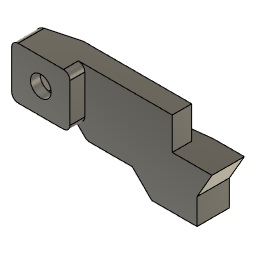
Omnivore adapter plate (Autodesk Fusion 360 design; units mm, degrees)
Autodesk Fusion 360 part; units mm, degrees
sketch "Sketch1" plane through (0, 0, 0) normal (0, 1, 0) x (1, 0, 0)
  line L0 (4.5, -4) -> (-4.5, -4)
  line L1 (-4.5, -4) -> (-4.5, 4)
  line L2 (-4.5, 4) -> (4.5, 4)
  line L3 (4.5, 4) -> (4.5, -4)
  line L4 (4.5, -4) -> (-4.5, 4) construction
  line L5 (-4.5, -4) -> (4.5, 4) construction
  dimension "d164" = 9
  dimension "d165" = 8
  constraint horizontal L0
  constraint perpendicular L0 L1
  constraint parallel L0 L2
  constraint parallel L1 L3
  constraint coincident L4 origin
  constraint coincident L5 origin
  measures "d164" distance of L1.end L2.end
  measures "d165" distance of L0.start L2.end
extrude "Extrude1" add sketch "Sketch1" along normal blind 2.3 makes body 1
fillet "Fillet1" radius 1 2 edges at (-4.5, 1.15, 4) (-4.5, 1.15, -4) on bodies 1
sketch "Sketch2" plane through (0, 2.3, 0) normal (0, 1, 0) x (-1, 0, 0)
  line L0 (-4.5, -4) -> (3.5, -4)
  arc A0 (3.5, -4) -> (4.5, -3) centre (3.5, -3) ccw
  line L1 (4.5, -3) -> (4.5, 3)
  arc A1 (4.5, 3) -> (3.5, 4) centre (3.5, 3) ccw
  line L2 (3.5, 4) -> (-4.5, 4)
  line L3 (-4.5, 4) -> (-4.5, -4)
  line L4 (-3.4641, 0) -> (-1.7321, -3)
  line L5 (-1.7321, -3) -> (1.7321, -3)
  line L6 (1.7321, -3) -> (3.4641, 0)
  line L7 (3.4641, 0) -> (1.7321, 3)
  line L8 (1.7321, 3) -> (-1.7321, 3)
  line L9 (-1.7321, 3) -> (-3.4641, 0)
  dimension "d170" = 6
  constraint horizontal L5
  measures "d170" distance of L4 L7
extrude "Extrude2" cut sketch "Sketch2" against normal up to surface (2.3 mm away) contours L4 L5 L6 L7 L8 L9 bodies 1
sketch "Sketch8" plane through (0, 2.3, 0) normal (0, 1, 0) x (-1, 0, 0)
  line L0 (-1.7321, -3) -> (-3.4641, 0)
  line L1 (-3.4641, 0) -> (-1.7321, 3)
  line L2 (-1.7321, 3) -> (1.7321, 3)
  line L3 (1.7321, 3) -> (3.4641, 0)
  line L4 (3.4641, 0) -> (1.7321, -3)
  line L5 (1.7321, -3) -> (-1.7321, -3)
  arc A0 (3.5, -4) -> (4.5, -3) centre (3.5, -3) ccw
  line L6 (4.5, -3) -> (4.5, 3)
  arc A1 (4.5, 3) -> (3.5, 4) centre (3.5, 3) ccw
  line L7 (3.5, 4) -> (-4.5, 4)
  line L8 (-4.5, 4) -> (-4.5, -4)
  line L9 (-4.5, -4) -> (3.5, -4)
extrude "Extrude6" add sketch "Sketch8" along normal blind 3 separate body makes body 2
sketch "Sketch19" plane through (0, 0, 0) normal (0, -1, 0) x (-1, 0, 0)
  line L0 (3.4641, 0) -> (1.7321, -3)
  line L1 (1.7321, -3) -> (-1.7321, -3)
  line L2 (-1.7321, -3) -> (-3.4641, 0)
  line L3 (-3.4641, 0) -> (-1.7321, 3)
  line L4 (-1.7321, 3) -> (1.7321, 3)
  line L5 (1.7321, 3) -> (3.4641, 0)
  line L6 (-4.5, -4) -> (3.5, -4)
  arc A0 (3.5, -4) -> (4.5, -3) centre (3.5, -3) ccw
  line L7 (4.5, -3) -> (4.5, 3)
  arc A1 (4.5, 3) -> (3.5, 4) centre (3.5, 3) ccw
  line L8 (3.5, 4) -> (-4.5, 4)
  line L9 (-4.5, 4) -> (-4.5, -4)
  line L10 (1.7321, -3) -> (3.4641, 0)
  line L11 (3.4641, 0) -> (1.7321, 3)
  line L12 (1.7321, 3) -> (-1.7321, 3)
  line L13 (-1.7321, 3) -> (-3.4641, 0)
  line L14 (-3.4641, 0) -> (-1.7321, -3)
  line L15 (-1.7321, -3) -> (1.7321, -3)
  circle A2 centre (0, 0) radius 1.6
  line L16 (3.4641, 0) -> (1.7321, -3)
  line L17 (1.7321, -3) -> (-1.7321, -3)
  line L18 (-1.7321, -3) -> (-3.4641, 0)
  line L19 (-3.4641, 0) -> (-1.7321, 3)
  line L20 (-1.7321, 3) -> (1.7321, 3)
  line L21 (1.7321, 3) -> (3.4641, 0)
  arc A3 (4.5, 3) -> (3.5, 4) centre (3.5, 3) ccw
  line L22 (3.5, 4) -> (-4.5, 4)
  line L23 (-4.5, 4) -> (-4.5, -4)
  line L24 (-4.5, -4) -> (3.5, -4)
  arc A4 (3.5, -4) -> (4.5, -3) centre (3.5, -3) ccw
  line L25 (4.5, -3) -> (4.5, 3)
  dimension "d231" = 3.2
  constraint collinear L4 L12
  constraint coincident L3.end L4.start
  constraint coincident L4.end L5.start
  constraint coincident A2.centre origin
  measures "d231" diameter of A2
extrude "Extrude14" add sketch "Sketch19" against normal blind 1.5 contours L0 L1 L2 L3 L4 L5 L10 L11 L12 L13 L14 L15 L16 L17 L18 L19 L20 L21 bodies 1
fillet "Fillet3" radius 1 2 edges at (4.5, 1.15, 4) (4.5, 1.15, -4) on bodies 1
sketch "Sketch11" plane through (4.5, 0, 0) normal (1, 0, 0) x (0, 1, 0)
  line L0 (2.3, 4) -> (2.3, -4)
  line L1 (2.3, -4) -> (5.3, -4)
  line L2 (5.3, -4) -> (5.3, 4)
  line L3 (5.3, 4) -> (2.3, 4)
extrude "Extrude7" add sketch "Sketch11" along normal blind 13.5 bodies 2 1
sketch "Sketch12" plane through (0, 0, -4) normal (0, 0, -1) x (1, 0, 0)
  line L0 (18, -2.3) -> (3.5, -2.3)
  line L1 (-3.5, 0) -> (-3.5, -5.3)
  line L2 (-3.5, -5.3) -> (18, -5.3)
  line L3 (18, -5.3) -> (18, -2.3)
  line L4 (18, -5.3) -> (2.83, -5.3)
  line L5 (2.83, -5.3) -> (2.83, -2.3)
  line L6 (2.83, -2.3) -> (18, -2.3)
  line L7 (18, -2.3) -> (18, -5.3)
  line L8 (3.5, -2.3) -> (3.5, 0)
  line L9 (3.5, 0) -> (-3.5, 0)
  line L10 (-4.5, 0) -> (-4.5, -5.3) construction
  dimension "d242" = 7.33
  constraint horizontal L4
  constraint vertical L5
  constraint horizontal L6
  constraint vertical L7
  constraint coincident L0 L5.end
  constraint coincident L2.end L3.start
  measures "d242" distance of L5 L10
extrude "Extrude8" add sketch "Sketch12" along normal blind 10 from surface at -8 contours L0 L2 L3 L4 L5 L6 L7 bodies 2
chamfer "Chamfer1" distance 2 angle 45 1 edges at (2.83, 3.8, -6) on bodies 2
fillet "Fillet6" radius 1 1 edges at (4.83, 3.8, -6) on bodies 2
ref_plane "WorkPlane1" through (18, 3.8, -6) normal (-0.707107, 0, 0.707107) x (0, -1, 0)
sketch "Sketch17" plane through (0, 5.3, 0) normal (0, 1, 0) x (-1, 0, 0)
  line L0 (-2.83, -4) -> (3.5, -4)
  arc A0 (3.5, -4) -> (4.5, -3) centre (3.5, -3) ccw
  line L1 (4.5, -3) -> (4.5, 3)
  arc A1 (4.5, 3) -> (3.5, 4) centre (3.5, 3) ccw
  line L2 (3.5, 4) -> (-18, 4)
  line L3 (-18, 4) -> (-18, -6)
  line L4 (-18, -6) -> (-5.2442, -6)
  line L5 (-4.5371, -5.7071) -> (-2.83, -4)
  line L6 (-18, -1) -> (-24.1394, -1)
  line L7 (-24.1394, -1) -> (-21.83, -5)
  line L8 (-21.83, -5) -> (-21.83, -9)
  line L9 (-21.83, -9) -> (-11.83, -9)
  line L10 (-11.83, -9) -> (-11.83, -6)
  arc A2 (-5.2442, -6) -> (-4.5371, -5.7071) centre (-5.2442, -5) ccw
  line L11 (-2.83, -1.0983) -> (-2.83, 1.0983) construction
  line L12 (-2.83, 1.0983) -> (-1.7321, 3) construction
  line L13 (-1.7321, 3) -> (1.7321, 3) construction
  line L14 (1.7321, 3) -> (3.4641, 0) construction
  line L15 (3.4641, 0) -> (1.7321, -3) construction
  line L16 (1.7321, -3) -> (-1.7321, -3) construction
  line L17 (-1.7321, -3) -> (-2.83, -1.0983) construction
  point P0 (-2.83, -4)
  dimension "d221" = 5
  dimension "d222" = 30
  dimension "d223" = 8
  dimension "d226" = 10
  dimension "d245" = 9
  dimension "d246" = 4
  constraint coincident L3 L6.start
  constraint coincident L4 L10.end
  constraint vertical L10
  constraint vertical L8
  constraint horizontal L9
  constraint horizontal L6
  measures "d221" distance of L2 L6
  measures "d222" angle of L7 L8
  measures "d223" distance of L6 L9
  measures "d226" distance of L8.end L9.end
  measures "d245" distance of L10 P0
  measures "d246" distance of L6 L7.end
extrude "Extrude12" add sketch "Sketch17" against normal up to surface (3 mm away) contours L3 L4 L6 L7 L8 L9 L10 bodies 2
chamfer "Chamfer2" distance 3 angle 45 1 edges at (11.83, 3.8, -9) on bodies 2
sketch "Sketch20" plane through (0, 5.3, 0) normal (0, 1, 0) x (1, 0, 0)
  line L0 (21.6394, 1) -> (19.33, 5)
  line L1 (19.33, 5) -> (19.33, 9)
  line L2 (18, 1) -> (24.1394, 1) construction
  line L3 (24.1394, 1) -> (21.83, 5) construction
  line L4 (19.33, 9) -> (21.83, 9)
  line L5 (21.83, 9) -> (14.83, 9) construction
  line L6 (21.83, 5) -> (21.83, 9) construction
  line L7 (24.1394, 1) -> (21.6394, 1)
  line L8 (21.83, 5) -> (21.83, 9)
  line L9 (21.83, 9) -> (21.83, 5)
  line L10 (21.83, 5) -> (24.1394, 1)
  dimension "d250" = 2.5
  constraint coincident L0.start L2
  constraint parallel L0 L3
  constraint vertical L1
  constraint horizontal L4
  constraint coincident L4.end L5.start
  constraint horizontal L0.end L3.end
  constraint coincident L2.end L3.start
  constraint parallel L2 L7
  constraint coincident L3.end L6.start
  measures "d250" distance of L1.end L4.end
extrude "Extrude16" add sketch "Sketch20" along normal blind 2 bodies 2
sketch "Sketch21" plane through (0, 0, -1) normal (0, 0, 1) x (-1, 0, 0)
  line L0 (-18, -2.3) -> (-24.1394, -2.3)
  line L1 (-24.1394, -2.3) -> (-24.1394, -7.3)
  line L2 (-24.1394, -7.3) -> (-21.6394, -7.3)
  line L3 (-21.6394, -7.3) -> (-21.6394, -5.3)
  line L4 (-21.6394, -5.3) -> (-18, -5.3)
  line L5 (-18, -5.3) -> (-18, -2.3)
  line L6 (-2.83, -5.3) -> (-19.33, -5.3)
  line L7 (-19.33, -5.3) -> (-19.33, -7.3)
  line L8 (-19.33, -7.3) -> (-2.83, -5.3)
  line L9 (-19.33, -5.3) -> (-19.33, -7.3) construction
  point P0 (-2.83, -5.3)
  constraint horizontal L6
  constraint vertical L7
  constraint collinear L7 L9
  constraint coincident L6.end L7.start
  constraint coincident L7.end L8.start
  constraint coincident P0 L6.start
extrude "Extrude17" add sketch "Sketch21" against normal up to surface (8 mm away) separate body contours L4 L6 L7 L8 makes body 3
sketch "Sketch23" plane through (19.33, 0, 0) normal (1, 0, 0) x (0, 1, 0)
  line L0 (5.3, -9) -> (7.3, -9)
  line L1 (7.3, -9) -> (7.3, -1)
  line L2 (7.3, -1) -> (5.3, -1)
  line L3 (5.3, -1) -> (5.3, -9)
  line L4 (5.3, -1) -> (7.3, -1)
  line L5 (5.3, -5) -> (7.3, -5)
  line L6 (5.3, -1) -> (5.3, -5)
  line L7 (7.3, -1) -> (7.3, -5)
  constraint coincident L2.end L3.start
  constraint coincident L5.start L6.end
  constraint coincident L1.end L2.start
  constraint coincident L5.end L7.end
extrude "Extrude18" add sketch "Sketch23" along normal up to surface contours L1 L2 L3 L4 L5 L6 L7 end surface through (21.6394, 5.3, -1) normal (-0.866025, 0, 0.5) offset 0 bodies 3
sketch "Sketch24" plane through (0, 5.3, 0) normal (0, -1, 0) x (1, 0, 0)
  line L0 (2.83, -9) -> (19.33, -9)
  line L1 (19.33, -9) -> (19.33, -5)
  line L2 (19.33, -5) -> (21.6394, -1)
  line L3 (21.6394, -1) -> (2.83, -1)
  line L4 (2.83, -1) -> (2.83, -9)
  line L5 (11.83, -6) -> (14.83, -9)
  line L6 (5.2442, -6) -> (11.83, -6)
  arc A0 (4.5371, -5.7071) -> (5.2442, -6) centre (5.2442, -5) ccw
  line L7 (2.83, -4) -> (4.5371, -5.7071)
  line L8 (14.83, -9) -> (2.83, -9)
  line L9 (2.83, -9) -> (2.83, -4)
  constraint coincident L5.end L8.start
  constraint coincident L0.start L4.end
  constraint coincident L7.start L9.end
extrude "Extrude19" cut sketch "Sketch24" along normal up to surface contours L0 L4 L5 L6 A0 L7 L8 L9 end surface through (19.33, 7.3, -1) normal (-0.120331, 0.992734, 0) offset 0 bodies 3
combine "Combine2" operation add target body 3 tool bodies 2
sketch "Sketch25" plane through (0, 0, 4) normal (0, 0, 1) x (-1, 0, 0)
  line L0 (-3.5, -2.3) -> (-18, -2.3)
  line L1 (-18, -2.3) -> (-18, -5.3)
  line L2 (-18, -5.3) -> (3.5, -5.3)
  line L3 (3.5, -5.3) -> (3.5, 0)
  line L4 (3.5, 0) -> (-3.5, 0)
  line L5 (-3.5, 0) -> (-3.5, -2.3)
  line L6 (4.5, -5.3) -> (-1.2956, -5.3)
  line L7 (-1.2956, -5.3) -> (4.5, -3.7471)
  line L8 (4.5, -3.7471) -> (4.5, -5.3)
  line L9 (4.5, 0) -> (4.5, -5.3)
  line L10 (-1.7321, -5.3) -> (1.7321, -5.3)
  dimension "d260" = 75
  dimension "d261" = 6
  constraint horizontal L6
  constraint vertical L8
  constraint collinear L8 L9
  constraint collinear L6 L10
  measures "d260" angle of L7 L8
  measures "d261" distance of L6.end L7.end
extrude "Extrude20" cut sketch "Sketch25" against normal up to surface (8 mm away) contours L3 L6 L7 L8 L9 | L2 L3 L6 L7 L10 bodies 3
equation "d222 = 30 °"
equation "d260 = 75 °"
